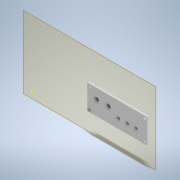
# Autodesk Inventor part: InterfacePlate
Saved by Autodesk Inventor 2022.2 (Build 262287000, 287)
## iProperties
Created: 2022-01-15
Part Number: InterfacePlate
Material: Generic
Document SubType Name: Modeling
Designer: siwat
Density: 1 g/cm^3
Appearance: Default
Author: siwat
Autodesk Inventor part; units mm, degrees
ref_plane "YZ Plane" through (0, 0, 0) normal (1, 0, 0) x (0, 1, 0)
ref_plane "XZ Plane" through (0, 0, 0) normal (0, 1, 0) x (-1, 0, 0)
ref_plane "XY Plane" through (0, 0, 0) normal (0, 0, 1) x (1, 0, 0)
ref_plane "Work Plane1" through (0, 0, 0) normal (0, 0, 1) x (1, 0, 0)
sketch "Sketch1" plane through (0, 0, 0) normal (0, 0, 1) x (1, 0, 0)
  line L0 (67.7271, 45.3897) -> (135.6749, 45.3897)
  line L1 (135.6749, 45.3897) -> (135.6749, 17.2701)
  line L2 (135.6749, 17.2701) -> (67.7271, 17.2701)
  line L3 (67.7271, 17.2701) -> (67.7271, 45.3897)
  circle A0 centre (70.3236, 42.7621) radius 1.5
  circle A1 centre (70.2655, 19.7679) radius 1.5
  circle A2 centre (132.8977, 19.6632) radius 1.5
  circle A3 centre (132.9442, 42.6673) radius 1.5
  point P0 (0, 0)
  dimension "d0" = 3
  dimension "d1" = 3
  dimension "d2" = 3
  dimension "d3" = 3
  constraints: 8 end point, 4 centre point, 2 parallel, 1 horizontal, 1 perpendicular
  measures "d0" diameter of A0
  measures "d1" diameter of A1
  measures "d2" diameter of A2
  measures "d3" diameter of A3
extrude "Extrusion1" add sketch "Sketch1" along normal blind 2
sketch "Sketch2" plane through (0, 0, 0) normal (0, 0, -1) x (-1, 0, 0)
  line L0 (-130.7904, 21.7727) -> (-72.4709, 21.7727)
  line L1 (-72.4709, 21.7727) -> (-72.4709, 40.605)
  line L2 (-72.4709, 40.605) -> (-130.7904, 40.605)
  line L3 (-130.7904, 40.605) -> (-130.7904, 21.7727)
  point P0 (0, 0)
  constraints: 8 end point, 2 parallel, 1 horizontal, 1 perpendicular
extrude "Extrusion2" add sketch "Sketch2" along normal blind 3
sketch "Sketch3" plane through (0, 0, -3) normal (0, 0, -1) x (-1, 0, 0)
  circle A0 centre (-123.1484, 27.6797) radius 1.75
  line L0 (-121.6186, 32.121) -> (-111.2555, 32.121)
  circle A1 centre (-113.1484, 27.6797) radius 1.75
  circle A2 centre (-103.1484, 27.6797) radius 1.75
  circle A3 centre (-91.5974, 33.7589) radius 2.5
  circle A4 centre (-78.3445, 33.7589) radius 2.5
  point P0 (0, 0)
  dimension "d8" = 3.5
  dimension "d11" = 10
  dimension "d16" = 5
  dimension "d17" = 5
  constraints: 5 centre point, 2 end point, 2 horizontal, 4 other
  measures "d8" diameter of A0
  measures "d11" distance of A0.centre A1.centre
  measures "d16" diameter of A3
  measures "d17" diameter of A4
extrude "Extrusion3" cut sketch "Sketch3" against normal up to surface (5 mm away)
sketch "Sketch4" plane through (0, 0, -3) normal (0, 0, -1) x (-1, 0, 0)
  line L0 (-126.3413, 33.4304) -> (-118.9387, 33.4304) construction
  line L1 (-118.9387, 33.4304) -> (-118.9387, 30.3319) construction
  line L2 (-118.9387, 30.3319) -> (-126.3413, 30.3319) construction
  line L3 (-126.3413, 30.3319) -> (-126.3413, 33.4304) construction
  line L4 (-116.3929, 33.3925) -> (-109.1583, 33.3925) construction
  line L5 (-109.1583, 33.3925) -> (-109.1583, 30.3319) construction
  line L6 (-109.1583, 30.3319) -> (-116.3929, 30.3319) construction
  line L7 (-116.3929, 30.3319) -> (-116.3929, 33.3925) construction
  line L8 (-107.7125, 33.476) -> (-98.1289, 33.476) construction
  line L9 (-98.1289, 33.476) -> (-98.1289, 30.3319) construction
  line L10 (-98.1289, 30.3319) -> (-107.7125, 30.3319) construction
  line L11 (-107.7125, 30.3319) -> (-107.7125, 33.476) construction
  line L12 (-95.4359, 29.1892) -> (-86.7439, 29.1892) construction
  line L13 (-86.7439, 29.1892) -> (-86.7439, 26.1412) construction
  line L14 (-86.7439, 26.1412) -> (-95.4359, 26.1412) construction
  line L15 (-95.4359, 26.1412) -> (-95.4359, 29.1892) construction
  line L16 (-80.7485, 29.2979) -> (-75.9197, 29.2979) construction
  line L17 (-75.9197, 29.2979) -> (-75.9197, 26.1412) construction
  line L18 (-75.9197, 26.1412) -> (-80.7485, 26.1412) construction
  line L19 (-80.7485, 26.1412) -> (-80.7485, 29.2979) construction
  point P0 (0, 0)
  constraints: 3 collinear, 10 other
body "Solid1"
